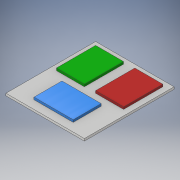
# Autodesk Inventor part: Stage with Boards
Saved by Autodesk Inventor 2018 (Build 220112000, 112)
## iProperties
Created: 2018-02-19
Part Number: Stage with Boards
Material: Generic
Document SubType Name: Modeling
Designer: Melda
Density: 1 g/cm^3
Appearance: Default
Author: Melda
Autodesk Inventor part; units mm, degrees
ref_plane "YZ Plane" through (0, 0, 0) normal (1, 0, 0) x (0, 1, 0)
ref_plane "XZ Plane" through (0, 0, 0) normal (0, 1, 0) x (-1, 0, 0)
ref_plane "XY Plane" through (0, 0, 0) normal (0, 0, 1) x (1, 0, 0)
sketch "Sketch1" plane through (0, 0, 0) normal (0, 1, 0) x (-1, 0, 0)
  line L0 (17.529, 129.5854) -> (-122.471, 129.5854)
  line L1 (-122.471, 129.5854) -> (-122.471, -30.4146)
  line L2 (-122.471, -30.4146) -> (17.529, -30.4146)
  line L3 (17.529, -30.4146) -> (17.529, 129.5854)
  point P0 (0, 0)
  dimension "d0" = 160
  dimension "d1" = 140
  constraints: 8 end point, 2 parallel, 1 horizontal, 1 perpendicular
  measures "d0" distance of L2.end L0.start
  measures "d1" distance of L1.end L2.end
extrude "Extrusion1" add sketch "Sketch1" along normal blind 4
sketch "Sketch2" plane through (0, 4, 0) normal (0, 1, 0) x (1, 0, 0)
  point P0 (0, 0)
sketch "Sketch3" plane through (0, 4, 0) normal (0, 1, 0) x (1, 0, 0)
  line L0 (17.471, -114.5854) -> (87.471, -114.5854)
  line L1 (87.471, -114.5854) -> (87.471, -64.5854)
  line L2 (87.471, -64.5854) -> (17.471, -64.5854)
  line L3 (17.471, -64.5854) -> (17.471, -114.5854)
  line L4 (-7.529, -49.5854) -> (42.471, -49.5854)
  line L5 (42.471, -49.5854) -> (42.471, 20.4146)
  line L6 (42.471, 20.4146) -> (-7.529, 20.4146)
  line L7 (-7.529, 20.4146) -> (-7.529, -49.5854)
  line L8 (62.471, -49.5854) -> (112.471, -49.5854)
  line L9 (112.471, -49.5854) -> (112.471, 20.4146)
  line L10 (112.471, 20.4146) -> (62.471, 20.4146)
  line L11 (62.471, 20.4146) -> (62.471, -49.5854)
  line L12 (-17.529, -129.5854) -> (122.471, -129.5854) projected
  line L13 (-17.529, 30.4146) -> (-17.529, -129.5854) projected
  line L14 (122.471, 30.4146) -> (-17.529, 30.4146) projected
  line L15 (122.471, -129.5854) -> (122.471, 30.4146) projected
  point P0 (0, 0)
  dimension "d4" = 50
  dimension "d5" = 70
  dimension "d6" = 50
  dimension "d7" = 50
  dimension "d8" = 70
  dimension "d9" = 70
  dimension "d10" = 15
  dimension "d11" = 10
  dimension "d12" = 10
  dimension "d13" = 10
  dimension "d14" = 10
  dimension "d15" = 35
  dimension "d16" = 35
  constraints: 24 end point, 6 parallel, 3 horizontal, 3 perpendicular
  measures "d4" distance of L2.end L0.start
  measures "d5" distance of L0.start L0.end
  measures "d6" distance of L5.end L6.end
  measures "d7" distance of L9.end L10.end
  measures "d8" distance of L6.end L4.start
  measures "d9" distance of L8.end L9.end
  measures "d10" distance between parallel lines of L12 L0
  measures "d11" distance between parallel lines of L13 L7
  measures "d12" distance between parallel lines of L14 L6
  measures "d13" distance between parallel lines of L14 L10
  measures "d14" distance between parallel lines of L15 L9
  measures "d15" distance between parallel lines of L3 L13
  measures "d16" distance between parallel lines of L15 L1
extrude "Extrusion2" add sketch "Sketch3" along normal blind 4 contours L3 L2 L1 L0 | L7 L6 L5 L4 | L11 L10 L9 L8
body "Solid1"
